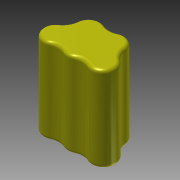
# Autodesk Inventor part: Battery Pack
Saved by Autodesk Inventor 2015 (Build 190159000, 159)
## iProperties
Created: 2015-01-26
Part Number: Battery Pack
Material: Generic
Document SubType Name: Modeling
Designer: Justin
Density: 1 g/cm^3
Appearance: Yellow
Author: Justin
Autodesk Inventor part; units mm, degrees
ref_plane "YZ Plane" through (0, 0, 0) normal (1, 0, 0) x (0, 1, 0)
ref_plane "XZ Plane" through (0, 0, 0) normal (0, 1, 0) x (-1, 0, 0)
ref_plane "XY Plane" through (0, 0, 0) normal (0, 0, 1) x (1, 0, 0)
sketch "Sketch1" plane through (0, 0, 0) normal (0, 0, 1) x (1, 0, 0)
  circle A0 centre (0, 0) radius 7.25
  circle A1 centre (14.5, 0) radius 7.25
  circle A2 centre (-7.25, -12.5574) radius 7.25
  circle A3 centre (7.25, -12.5574) radius 7.25
  circle A4 centre (21.75, -12.5574) radius 7.25
  dimension "d0" = 14.5
  dimension "d1" = 14.5
  dimension "d2" = 14.5
  dimension "d3" = 14.5
  dimension "d4" = 14.5
  dimension "d5" = 14.5
  constraints: 6 equal radius, 5 centre point, 1 coincident, 1 horizontal alignment
  measures "d0" diameter of A0
  measures "d1" diameter of A1
  measures "d2" distance of point (0, 0) A1.centre
  measures "d3" diameter of A3
  measures "d4" diameter of A2
  measures "d5" diameter of A4
extrude "Extrusion1" add sketch "Sketch1" along normal blind 51.65 contours A0 | A1 | A2 | A3 | A4
sketch "Sketch2" plane through (0, 0, 51.65) normal (0, 0, 1) x (1, 0, 0)
  arc A0 (18.125, -6.2787) -> (7.25, 0) centre (14.5, 0) ccw projected
  arc A1 (14.5, -12.5574) -> (10.875, -6.2787) centre (7.25, -12.5574) ccw projected
  arc A2 (10.875, -6.2787) -> (3.625, -6.2787) centre (7.25, -12.5574) ccw projected
  arc A3 (3.625, -6.2787) -> (0, -12.5574) centre (7.25, -12.5574) ccw projected
  arc A4 (0, -12.5574) -> (14.5, -12.5574) centre (7.25, -12.5574) ccw projected
  arc A5 (0, -12.5574) -> (-3.625, -6.2787) centre (-7.25, -12.5574) ccw projected
  arc A6 (-3.625, -6.2787) -> (0, -12.5574) centre (-7.25, -12.5574) ccw projected
  arc A7 (14.5, -12.5574) -> (18.125, -6.2787) centre (21.75, -12.5574) ccw projected
  arc A8 (18.125, -6.2787) -> (14.5, -12.5574) centre (21.75, -12.5574) ccw projected
  arc A9 (7.25, 0) -> (-3.625, -6.2787) centre (0, 0) ccw projected
  arc A10 (-3.625, -6.2787) -> (3.625, -6.2787) centre (0, 0) ccw projected
  arc A11 (3.625, -6.2787) -> (7.25, 0) centre (0, 0) ccw projected
  line L0 (-1, 1) -> (15.5, 1)
  line L1 (15.5, 1) -> (22.75, -13.5574)
  line L2 (22.75, -13.5574) -> (-8.25, -13.5574)
  arc A12 (-3.625, -6.2787) -> (0, -12.5574) centre (-7.25, -12.5574) ccw projected
  line L3 (-1, 1) -> (-8.25, -13.5574)
  dimension "d8" = 1
  dimension "d9" = 1
  dimension "d10" = 1
  dimension "d11" = 1
  dimension "d12" = 1
  dimension "d13" = 1
  constraints: 8 end point, 1 horizontal, 1 horizontal alignment
  measures "d8" horizontal distance of A5.centre L2.end
  measures "d9" horizontal distance of A5.centre L2.end
  measures "d10" horizontal distance of A7.centre L1.end
  measures "d11" distance from line of L0 A0.centre
  measures "d12" horizontal distance of L0.end A0.centre
  measures "d13" horizontal distance of L0.start point (0, 0)
extrude "Extrusion2" add sketch "Sketch2" against normal blind 51.65 contours A8 A1 A2 A11 A0 L0 L1 | A0 L1 A7 | A7 L1 L2 A8 | A4 L2 A3 A2 A1 | A7 L2 A4 | A0 A9 L0 | A11 A10 A9 L3 L0 | A3 A5 A10 | L2 A6 A4 | A9 A6 L3 | A6 L2 L3 A5
fillet "Fillet1" radius 10 10 edges at (7.1807, 1, 25.825) (7.3193, 1, 25.825) (-4.3766, -5.7799, 25.825) (-4.4264, -5.8798, 25.825) (-0.0693, -13.5574, 25.825) (0.0693, -13.5574, 25.825) (14.4307, -13.5574, 25.825) (14.5693, -13.5574, 25.825) (18.8766, -5.7799, 25.825) (18.9264, -5.8798, 25.825)
fillet "Fillet2" radius 2 20 edges at (18.125, 6.2787, 51.65) (23.0202, -3.4524, 51.65) (28.0287, -16.1824, 51.65) (14.5, -18.2098, 51.65) (7.25, -19.8074, 51.65) (0, -18.2098, 51.65) (-13.5287, -16.1824, 51.65) (-8.5202, -3.4524, 51.65) (-3.625, 6.2787, 51.65) (7.25, 5.6525, 51.65) (23.0202, -3.4524, 0) (28.0287, -16.1824, 0) (14.5, -18.2098, 0) (7.25, -19.8074, 0) (0, -18.2098, 0) (-13.5287, -16.1824, 0) (-8.5202, -3.4524, 0) (-3.625, 6.2787, 0) (7.25, 5.6525, 0) (18.125, 6.2787, 0)
body "Solid1"
